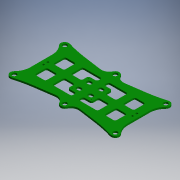
# Autodesk Inventor part: Body_bottom
Saved by Autodesk Inventor 2017 (Build 210142000, 142)
## iProperties
Part Number: Body_bottom
Material: Generic
Document SubType Name: Modeling
Designer: alex-
Appearance: Dark Green
b_mat_thickness: 0,500 cm
b_core_width: 15,000 cm
b_leg_space: 15,000 cm
Author: alex-
Autodesk Inventor part; units mm, degrees
ref_plane "YZ Plane" through (0, 0, 0) normal (1, 0, 0) x (0, 1, 0)
ref_plane "XZ Plane" through (0, 0, 0) normal (0, 1, 0) x (-1, 0, 0)
ref_plane "XY Plane" through (0, 0, 0) normal (0, 0, 1) x (1, 0, 0)
sketch "Sketch1" plane through (0, 0, 0) normal (0, 1, 0) x (-1, 0, 0)
  line L0 (166.0997, -69.6334) -> (155.3666, -91.0997)
  line L1 (155.3666, -91.0997) -> (133.9003, -80.3666)
  line L2 (133.9003, -80.3666) -> (144.6334, -58.9003) construction
  line L3 (144.6334, -58.9003) -> (166.0997, -69.6334)
  line L4 (144.6334, -58.9003) -> (155.3666, -91.0997) construction
  line L5 (12, -87) -> (-12, -87)
  line L6 (-12, -87) -> (-12, -63)
  line L7 (-12, -63) -> (12, -63) construction
  line L8 (12, -63) -> (12, -87)
  line L9 (12, -63) -> (-12, -87) construction
  line L10 (-155.3666, -91.0997) -> (-166.0997, -69.6334)
  line L11 (-166.0997, -69.6334) -> (-144.6334, -58.9003)
  line L12 (-144.6334, -58.9003) -> (-133.9003, -80.3666) construction
  line L13 (-133.9003, -80.3666) -> (-155.3666, -91.0997)
  line L14 (-133.9003, -80.3666) -> (-166.0997, -69.6334) construction
  line L15 (155.3666, 91.0997) -> (166.0997, 69.6334)
  line L16 (166.0997, 69.6334) -> (144.6334, 58.9003)
  line L17 (144.6334, 58.9003) -> (133.9003, 80.3666) construction
  line L18 (133.9003, 80.3666) -> (155.3666, 91.0997)
  line L19 (133.9003, 80.3666) -> (166.0997, 69.6334) construction
  line L20 (12, 63) -> (-12, 63) construction
  line L21 (-12, 63) -> (-12, 87)
  line L22 (-12, 87) -> (12, 87)
  line L23 (12, 87) -> (12, 63)
  line L24 (12, 87) -> (-12, 63) construction
  line L25 (-166.0997, 69.6334) -> (-155.3666, 91.0997)
  line L26 (-155.3666, 91.0997) -> (-133.9003, 80.3666)
  line L27 (-133.9003, 80.3666) -> (-144.6334, 58.9003) construction
  line L28 (-144.6334, 58.9003) -> (-166.0997, 69.6334)
  line L29 (-144.6334, 58.9003) -> (-155.3666, 91.0997) construction
  line L30 (160.7331, -80.3666) -> (-160.7331, -80.3666) construction
  line L31 (-160.7331, -80.3666) -> (-160.7331, 80.3666) construction
  line L32 (-160.7331, 80.3666) -> (160.7331, 80.3666) construction
  line L33 (160.7331, 80.3666) -> (160.7331, -80.3666) construction
  line L34 (160.7331, -80.3666) -> (-160.7331, 80.3666) construction
  line L35 (160.7331, 80.3666) -> (-160.7331, -80.3666) construction
  line L36 (133.9003, 80.3666) -> (12, 63)
  line L37 (-12, 63) -> (-133.9003, 80.3666)
  line L38 (-144.6334, 58.9003) -> (-144.6334, -58.9003)
  line L39 (-133.9003, -80.3666) -> (-12, -63)
  line L40 (12, -63) -> (133.9003, -80.3666)
  line L41 (144.6334, -58.9003) -> (144.6334, 58.9003)
  point P0 (0, 0)
  point P1 (0, 0)
  point P2 (144.6334, -85.7331)
  point P3 (144.6334, 85.7331)
  point P4 (0, 0)
  point P5 (0, -75)
  point P6 (150, -75)
  point P7 (0, 75)
  point P8 (150, 75)
  point P9 (-150, 75)
  dimension "d27" = 24
  dimension "d28" = 24
  dimension "d30" = 24
  dimension "d32" = 24
  dimension "d34" = 24
  dimension "d36" = 24
  dimension "d40" = 150
  dimension "d42" = 150
  constraints: 84 end point, 17 perpendicular, 15 parallel, 13 midpoint, 2 horizontal, 2 horizontal alignment, 2 vertical alignment, 1 coincident, 1 point on line
  measures "d27" distance of L0.start L0.end
  measures "d28" distance of L5.start L5.end
  measures "d30" distance of L10.start L10.end
  measures "d32" distance of L15.start L15.end
  measures "d34" distance of L20.start L20.end
  measures "d36" distance of L25.start L25.end
  measures "d40" distance of point (150, -75) point (150, 75)
  measures "d42" distance of point (0, 75) point (150, 75)
extrude "Extrusion1" add sketch "Sketch1" along normal blind 5
fillet "Fillet3" radius 12 12 edges at (-155.3666, 2.5, 91.0997) (-166.0997, 2.5, 69.6334) (-166.0997, 2.5, -69.6334) (-155.3666, 2.5, -91.0997) (-12, 2.5, -87) (12, 2.5, -87) (155.3666, 2.5, -91.0997) (166.0997, 2.5, -69.6334) (166.0997, 2.5, 69.6334) (155.3666, 2.5, 91.0997) (12, 2.5, 87) (-12, 2.5, 87)
fillet "Fillet4" radius 24 4 edges at (-12, 2.5, 63) (12, 2.5, 63) (-12, 2.5, -63) (12, 2.5, -63)
fillet "Fillet5" radius 360 4 edges at (-133.9003, 2.5, 80.3666) (133.9003, 2.5, 80.3666) (133.9003, 2.5, -80.3666) (-133.9003, 2.5, -80.3666)
fillet "Fillet6" radius 48 4 edges at (-144.6334, 2.5, 58.9003) (-144.6334, 2.5, -58.9003) (144.6334, 2.5, -58.9003) (144.6334, 2.5, 58.9003)
sketch "Sketch5" plane through (0, 5, 0) normal (0, 1, 0) x (1, 0, 0)
  line L0 (-119.6334, 45) -> (119.6334, 45)
  line L1 (119.6334, 45) -> (119.6334, -45)
  line L2 (119.6334, -45) -> (-119.6334, -45)
  line L3 (-119.6334, -45) -> (-119.6334, 45)
  line L4 (-144.6334, 32.7816) -> (-144.6334, -32.7816) construction
  arc A0 (10.8805, 80.061) -> (-10.8805, 80.061) centre (0, 75) ccw construction
  line L5 (-35, 30.75) -> (35, 30.75)
  line L6 (35, 30.75) -> (35, -30.75)
  line L7 (35, -30.75) -> (-35, -30.75)
  line L8 (-35, -30.75) -> (-35, 30.75)
  line L9 (-25, 20.75) -> (25, 20.75)
  line L10 (25, 20.75) -> (25, -20.75)
  line L11 (25, -20.75) -> (-25, -20.75)
  line L12 (-25, -20.75) -> (-25, 20.75)
  line L13 (-25, 10) -> (-10, 10)
  line L14 (-10, 10) -> (-10, 20.75)
  line L15 (10, 20.75) -> (10, 10)
  line L16 (10, 10) -> (25, 10)
  line L17 (25, -10) -> (10, -10)
  line L18 (10, -10) -> (10, -20.75)
  line L19 (-25, -10) -> (-10, -10)
  line L20 (-10, -10) -> (-10, -20.75)
  line L21 (-35, -10) -> (-119.6334, -10)
  line L22 (-35, 10) -> (-119.6334, 10)
  line L23 (35, 10) -> (119.6334, 10)
  line L24 (35, -10) -> (119.6334, -10)
  line L25 (-226.8, 0) -> (226.8, 0) construction
  line L26 (0, 121.8) -> (0, -121.8) construction
  line L27 (-10, 30.75) -> (-10, 45)
  line L28 (10, 30.75) -> (10, 45)
  line L29 (-10, -30.75) -> (-10, -45)
  line L30 (10, -30.75) -> (10, -45)
  line L31 (-87.3167, 45) -> (-87.3167, 10)
  line L32 (-67.3167, 45) -> (-67.3167, 10)
  line L33 (-87.3167, -10) -> (-87.3167, -45)
  line L34 (-67.3167, -10) -> (-67.3167, -45)
  line L35 (67.3167, 45) -> (67.3167, 10)
  line L36 (87.3167, 45) -> (87.3167, 10)
  line L37 (67.3167, -10) -> (67.3167, -45)
  line L38 (87.3167, -10) -> (87.3167, -45)
  line L39 (-87.3167, 27.5) -> (-67.3167, 27.5) construction
  line L40 (-77.3167, 27.5) -> (-77.3167, 20) construction
  circle A1 centre (-29, 24.5) radius 1.375
  circle A2 centre (29, 24.5) radius 1.375
  circle A3 centre (-29, -24.5) radius 1.375
  circle A4 centre (29, -24.5) radius 1.375
  point P0 (0, 0)
  point P1 (0, 45)
  point P2 (-119.6334, 0)
  point P3 (0, 30.75)
  point P4 (35, 0)
  point P5 (0, 20.75)
  point P6 (-25, 0)
  point P7 (1.6129, 86.8911)
  point P8 (-1.6129, 86.8911)
  dimension "d47" = 25
  dimension "d48" = 30
  dimension "d49" = 70
  dimension "d50" = 61.5
  dimension "d51" = 10
  dimension "d52" = 10
  dimension "d53" = 20
  dimension "d54" = 20
  dimension "d55" = 20
  dimension "d56" = 20
  dimension "d63" = 2.75
  dimension "d64" = 29
  dimension "d65" = 24.5
  constraints: 74 end point, 54 point on line, 11 parallel, 11 perpendicular, 10 horizontal alignment, 8 midpoint, 6 vertical alignment, 4 centre point, 3 horizontal, 3 symmetric about line, 3 vertical, 17 other
  measures "d47" distance between parallel lines of L4 L3
  measures "d49" distance of L5.start L5.end
  measures "d50" distance of L5.end L6.end
  measures "d51" distance between parallel lines of L8 L12
  measures "d52" distance between parallel lines of L5 L9
  measures "d53" distance between parallel lines of L23 L24
  measures "d54" distance between parallel lines of L28 L27
  measures "d55" distance between parallel lines of L32 L31
  measures "d56" distance between parallel lines of L36 L35
  measures "d63" diameter of A1
  measures "d64" distance from line of L26 A1.centre
  measures "d65" distance from line of L25 A1.centre
extrude "Extrusion3" cut sketch "Sketch5" against normal up to next contours L0 L31 L22 L3 | L0 L27 L5 L8 L22 L32 | L21 L33 L2 L3 | L0 L35 L23 L6 L5 L28 | L21 L8 L7 L29 L2 L34 | L0 L1 L23 L36 | L30 L7 L6 L24 L37 L2 | L1 L2 L38 L24 | L9 L14 L13 L12 | L9 L10 L16 L15 | L19 L20 L11 L12 | L10 L11 L18 L17 | A1 | A2 | A3 | A4
fillet "Fillet7" radius 5 56 edges at (-119.6334, 2.5, -45) (-87.3167, 2.5, -45) (-87.3167, 2.5, -10) (-119.6334, 2.5, -10) (-119.6334, 2.5, 10) (-87.3167, 2.5, 10) (-119.6334, 2.5, 45) (-87.3167, 2.5, 45) (-67.3167, 2.5, 45) (-67.3167, 2.5, 10) (-35, 2.5, 10) (-35, 2.5, 30.75) (-10, 2.5, 30.75) (-10, 2.5, 45) (-10, 2.5, 20.75) (-10, 2.5, 10) (-25, 2.5, 10) (-25, 2.5, 20.75) (-25, 2.5, -20.75) (-25, 2.5, -10) (-10, 2.5, -10) (-10, 2.5, -20.75) (10, 2.5, -20.75) (10, 2.5, -10) (25, 2.5, -10) (25, 2.5, -20.75) (-10, 2.5, -30.75) (-10, 2.5, -45) (-67.3167, 2.5, -45) (-67.3167, 2.5, -10) (-35, 2.5, -10) (10, 2.5, 10) (10, 2.5, 20.75) (25, 2.5, 20.75) (25, 2.5, 10) (10, 2.5, -45) (10, 2.5, -30.75) (67.3167, 2.5, -45) (35, 2.5, -30.75) (35, 2.5, -10) (67.3167, 2.5, -10) (87.3167, 2.5, -45) (119.6334, 2.5, -45) (119.6334, 2.5, -10) (87.3167, 2.5, -10) (87.3167, 2.5, 10) (119.6334, 2.5, 10) (119.6334, 2.5, 45) (87.3167, 2.5, 45) (35, 2.5, 10) (67.3167, 2.5, 10) (67.3167, 2.5, 45) (10, 2.5, 45) (10, 2.5, 30.75) (35, 2.5, 30.75) (-35, 2.5, -30.75)
sketch "Sketch6" plane through (0, 5, 0) normal (0, 1, 0) x (1, 0, 0)
  circle A0 centre (-150, 75) radius 6.5
  circle A1 centre (0, 75) radius 6.5
  circle A2 centre (150, 75) radius 6.5
  circle A3 centre (150, -75) radius 6.5
  circle A4 centre (0, -75) radius 6.5
  circle A5 centre (-150, -75) radius 6.5
  arc A6 (-146.5024, 86.479) -> (-158.5267, 66.5563) centre (-150, 75) ccw projected
  arc A7 (10.8805, 80.061) -> (-10.8805, 80.061) centre (0, 75) ccw projected
  arc A8 (158.5267, 66.5563) -> (146.5024, 86.479) centre (150, 75) ccw projected
  arc A9 (146.5024, -86.479) -> (158.5267, -66.5563) centre (150, -75) ccw projected
  arc A10 (-10.8805, -80.061) -> (10.8805, -80.061) centre (0, -75) ccw projected
  arc A11 (-158.5267, -66.5563) -> (-146.5024, -86.479) centre (-150, -75) ccw projected
  point P0 (0, 0)
  point P1 (1.6129, 86.8911)
  point P2 (-1.6129, 86.8911)
  point P3 (-1.6129, -86.8911)
  point P4 (1.6129, -86.8911)
  dimension "d60" = 13
  constraints: 6 centre point, 6 concentric, 5 equal radius
  measures "d60" diameter of A0
extrude "Extrusion4" cut sketch "Sketch6" against normal up to next
sketch "Sketch7" plane through (0, 5, 0) normal (0, 1, 0) x (1, 0, 0)
  line L0 (-226.8, 0) -> (226.8, 0) construction
  line L1 (0, 121.8) -> (0, -121.8) construction
  line L2 (-134.6334, 9) -> (-129.6334, 9)
  line L3 (-129.6334, 9) -> (-129.6334, 4)
  line L4 (-129.6334, 4) -> (-134.6334, 4)
  line L5 (-134.6334, 4) -> (-134.6334, 9)
  line L6 (-144.6334, 32.7816) -> (-144.6334, -32.7816) projected
  line L7 (-134.6334, -9) -> (-129.6334, -9)
  line L8 (-129.6334, -9) -> (-129.6334, -4)
  line L9 (-129.6334, -4) -> (-134.6334, -4)
  line L10 (-134.6334, -4) -> (-134.6334, -9)
  line L11 (134.6334, 9) -> (129.6334, 9)
  line L12 (129.6334, 9) -> (129.6334, 4)
  line L13 (129.6334, 4) -> (134.6334, 4)
  line L14 (134.6334, 4) -> (134.6334, 9)
  line L15 (134.6334, -9) -> (129.6334, -9)
  line L16 (129.6334, -9) -> (129.6334, -4)
  line L17 (129.6334, -4) -> (134.6334, -4)
  line L18 (134.6334, -4) -> (134.6334, -9)
  point P0 (0, 0)
  dimension "d66" = 10
  dimension "d67" = 4
  dimension "d68" = 5
  constraints: 32 end point, 12 symmetric about line, 2 parallel, 2 perpendicular, 1 horizontal
  measures "d66" distance between parallel lines of L5 L6
  measures "d67" distance between parallel lines of L0 L4
  measures "d68" distance of L2.start L2.end
extrude "Extrusion5" cut sketch "Sketch7" against normal up to next
equation "\"d27\" = sa_diameter"
equation "\"d28\" = d29"
equation "\"d30\" = d31"
equation "\"d32\" = d33"
equation "\"d34\" = d35"
equation "\"d36\" = d37"
equation "\"d6\" = b_mat_thickness"
equation "\"b_mat_thickness\" = 5"
equation "\"b_core_width\" = 150"
equation "\"b_leg_space\" = 150"
equation "\"sa_diameter\" = 24"
equation "\"d29\" = 24"
equation "\"d31\" = 24"
equation "\"d33\" = 24"
equation "\"d35\" = 24"
equation "\"d37\" = 24"
body "Solid1"
